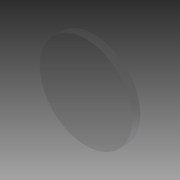
# Autodesk Inventor part: cam.case.glass
Saved by Autodesk Inventor 2011 (Build 150239000, 239)
## iProperties
Created: 2011-03-23
Part Number: cam.case.glass
Material: Glass
Document SubType Name: Modeling
Designer: Rob
Mass: 5.81798 g
Surface Area: 23.9328 cm^2
Volume: 2.6688 cm^3
Density: 2.18 g/cm^3
Author: Rob
Autodesk Inventor part; units mm, degrees
ref_plane "YZ Plane" through (0, 0, 0) normal (1, 0, 0) x (0, 1, 0)
ref_plane "XZ Plane" through (0, 0, 0) normal (0, 1, 0) x (-1, 0, 0)
ref_plane "XY Plane" through (0, 0, 0) normal (0, 0, 1) x (1, 0, 0)
sketch "Sketch1" plane through (0, 0, 0) normal (0, 0, 1) x (1, 0, 0)
  circle A0 centre (0, 0) radius 18.288
  dimension "d0" = 36.576
  dimension "d0" = 36.576
  constraints: 1 centre point, 1 coincident
  measures "d0" diameter of A0
extrude "Extrusion1" add sketch "Sketch1" along normal blind 3.175
body "Solid1"
